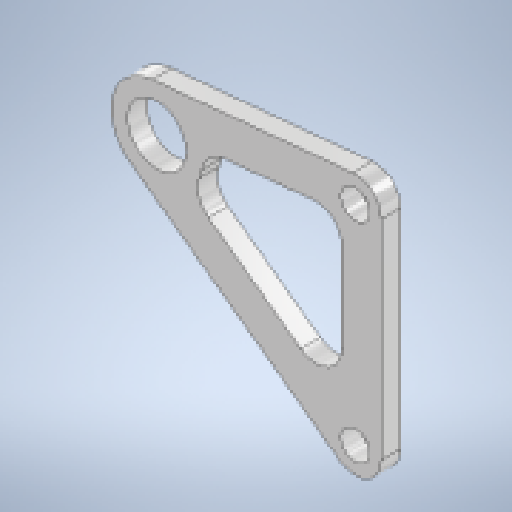
# Autodesk Inventor part: servolink
Saved by Autodesk Inventor 2025.1 (Build 291241000, 241)
## iProperties
Created: 2024-09-02
Part Number: servolink
Material: アルミニウム 2014-T4
Document SubType Name: Modeling
Designer: right
Density: 2.8 g/cm^3
Appearance: サテン
Mass: 0.554814 g
Surface Area: 4.83008 cm^2
Volume: 0.198148 cm^3
Author: right
Autodesk Inventor part; units mm, degrees
ref_plane "YZ Plane" through (0, 0, 0) normal (1, 0, 0) x (0, 1, 0)
ref_plane "XZ Plane" through (0, 0, 0) normal (0, 1, 0) x (-1, 0, 0)
ref_plane "XY Plane" through (0, 0, 0) normal (0, 0, 1) x (1, 0, 0)
sketch "スケッチ1" plane through (0, 0, 0) normal (0, 0, 1) x (1, 0, 0)
  line L0 (-18, -8) -> (18, -8) construction
  line L1 (18, -8) -> (18, 8) construction
  line L2 (18, 8) -> (-18, 8) construction
  line L3 (-18, 8) -> (-18, -8) construction
  line L4 (-18, -8) -> (18, 8) construction
  line L5 (18, -8) -> (-18, 8) construction
  circle A0 centre (-18, 8) radius 1.1
  circle A1 centre (18, 8) radius 1.1
  circle A2 centre (-18, -8) radius 1.1
  circle A3 centre (18, -8) radius 1.1
  circle A4 centre (-18, 8) radius 2
  circle A5 centre (-18, -8) radius 2
  line L6 (-16, 8) -> (-16, -8)
  circle A6 centre (-35.2333, 5) radius 2.25
  circle A7 centre (-35.2333, 5) radius 3.5
  line L7 (-35.5357, 8.4869) -> (-18.1728, 9.9925)
  line L8 (-37.1418, 2.0661) -> (-19.0906, -9.6765)
  circle A8 centre (11.5, 0) radius 8 projected
  line L9 (-35.2333, 5) -> (11.5, 0) construction
  point P0 (0, 0)
  point P1 (-16, 0)
  dimension "d0" = 36
  dimension "d1" = 16
  dimension "d2" = 2.2
  dimension "d5" = 36
  dimension "d8" = 16
  dimension "d11" = 4
  dimension "d12" = 4
  dimension "d13" = 4.5
  dimension "d14" = 7
  dimension "d16" = 5
  dimension "d19" = 47
  constraints: 20 end point, 8 centre point, 6 point on circle, 5 tangent, 4 coincident, 3 midpoint, 2 horizontal, 2 parallel, 2 perpendicular, 1 point on line, 1 vertical, 6 other
  measures "d0" distance of L1.end L2.end
  measures "d1" distance of L0.end L1.end
  measures "d2" diameter of A0
  measures "d5" distance of A0.centre A1.centre
  measures "d8" distance of A0.centre A2.centre
  measures "d11" diameter of A4
  measures "d12" diameter of A5
  measures "d13" diameter of A6
  measures "d14" diameter of A7
  measures "d16" vertical distance of point (-16, 0) A6.centre
  measures "d19" distance of L9.start L9.end
extrude "押し出し1" add sketch "スケッチ1" along normal blind 1.5 contours A4 | L6 A5 L8 A7 L7 A4 | A5 | A7
sketch "スケッチ2" plane through (0, 0, 0) normal (0, 0, -1) x (-1, 0, 0)
  line L0 (37.1418, 2.0661) -> (19.0906, -9.6765) projected
  arc A0 (37.1418, 2.0661) -> (35.5357, 8.4869) centre (35.2333, 5) ccw projected
  line L1 (18.1728, 9.9925) -> (35.5357, 8.4869) projected
  arc A1 (18.1728, 9.9925) -> (16, 8) centre (18, 8) ccw projected
  line L2 (16, -8) -> (16, 8) projected
  arc A2 (16, -8) -> (19.0906, -9.6765) centre (18, -8) ccw projected
  circle A3 centre (18, -8) radius 1.1 projected
  circle A4 centre (18, 8) radius 1.1 projected
  circle A5 centre (35.2333, 5) radius 2.25 projected
  line L3 (18, -8) -> (36.0512, 3.7426)
  arc A6 (36.0512, 3.7426) -> (35.3629, 6.4944) centre (35.2333, 5) ccw
  line L4 (35.3629, 6.4944) -> (18, 8)
  line L5 (18, 8) -> (18, -8)
  circle A7 centre (18, 8) radius 2
  circle A8 centre (18, -8) radius 2
  circle A9 centre (35.2333, 5) radius 3.5
  point P0 (0, 0)
  point P1 (33.4005, 2.0183)
  point P2 (32.2124, 6.7676)
  point P3 (19.9925, 7.8272)
  point P4 (18, 6)
  point P5 (33.6921, 6.6393)
  point P6 (34.6454, 2.8281)
  point P7 (20, 7.9971)
  point P8 (18.4708, 6.0562)
  point P9 (19, 2.9103)
  point P10 (18, -6.9)
  point P11 (18.9221, -7.4002)
  point P12 (18, -6)
  point P13 (19.6765, -6.9094)
  point P14 (18, 6.9)
  point P15 (19.0959, 7.905)
  dimension "d20" = 2
  constraints: 6 end point, 3 coincident, 2 centre point, 2 point on circle, 1 tangent, 10 other
  measures "d20" distance between parallel lines of L0 L3
extrude "押し出し2" cut sketch "スケッチ2" against normal through all contours L3 A8 L5 A7 L4 A9 | A5 L4 A6 L3 | L3 L5 A3 | A4 L5 L4 picked at (34.8052, 4.9839) picked at (18.0902, -7.2779) picked at (18.7117, 7.8482)
fillet "フィレット1" radius 2 6 edges at (-33.4005, 2.0183, 0.75) (-32.2124, 6.7676, 0.75) (-18, -6, 0.75) (-19.6765, -6.9094, 0.75) (-18, 6, 0.75) (-19.9925, 7.8272, 0.75)
equation "\"d5\" = d0"
equation "\"d8\" = d1"
